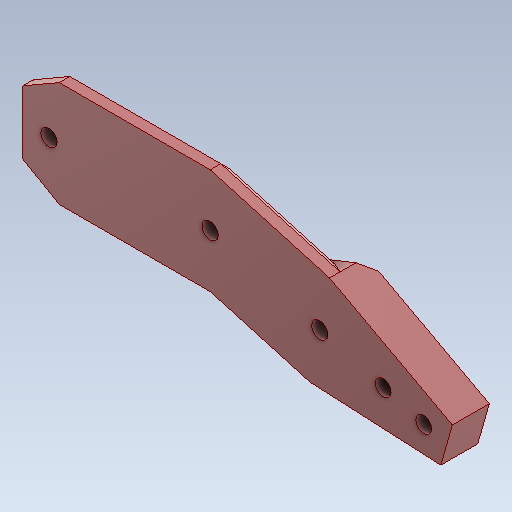
# Autodesk Inventor part: Fibula
Saved by Autodesk Inventor 2020 (Build 240168000, 168)
## iProperties
Created: 2020-09-15
Part Number: Fibula
Material: Generic
Document SubType Name: Modeling
Designer: Turing
Density: 1 g/cm^3
Appearance: Smooth - Burnt Red
Mass: 6.79509 g
Surface Area: 41.4305 cm^2
Volume: 6.79509 cm^3
Author: Turing
Autodesk Inventor part; units mm, degrees
ref_plane "YZ Plane" through (0, 0, 0) normal (1, 0, 0) x (0, 1, 0)
ref_plane "XZ Plane" through (0, 0, 0) normal (0, 1, 0) x (-1, 0, 0)
ref_plane "XY Plane" through (0, 0, 0) normal (0, 0, 1) x (1, 0, 0)
sketch "Sketch1" plane through (0, 0, 0) normal (0, 0, 1) x (1, 0, 0)
  circle A0 centre (0, 0) radius 1.55
  line L0 (0, 0) -> (30.548, 0)
  circle A1 centre (30.548, 0) radius 1.55
  line L1 (30.548, 0) -> (51.3166, -5.9278)
  circle A2 centre (51.3166, -5.9278) radius 1.55
  line L2 (0, 0) -> (-5, 0)
  line L3 (-5, 0) -> (-5, 6)
  line L4 (-5, 6) -> (1.9282, 10)
  line L5 (-5, 0) -> (-5, -6)
  line L6 (1.9282, 10) -> (30.548, 10)
  line L7 (-5, -6) -> (1.9282, -10)
  line L8 (1.9282, -10) -> (30.548, -10)
  line L9 (30.548, -10) -> (49.4624, -15.3986)
  line L10 (30.548, 10) -> (53.1707, 3.5429)
  line L11 (0, 0) -> (1.9282, 0)
  line L12 (51.3166, -5.9278) -> (75.3565, -12.7894)
  line L13 (75.3565, -12.7894) -> (76.4544, -8.943)
  line L14 (76.4544, -8.943) -> (53.1707, 3.5429)
  line L15 (75.3565, -12.7894) -> (74.2587, -16.6358)
  line L16 (49.4624, -15.3986) -> (74.2587, -16.6358)
  line L17 (51.3166, -5.9278) -> (75.3565, -12.7894)
  circle A3 centre (63.3366, -9.3586) radius 1.5
  line L18 (63.3366, -9.3586) -> (71.0293, -11.5543)
  circle A4 centre (71.0293, -11.5543) radius 1.5
  dimension "d0" = 3.1
  dimension "d1" = 30.548
  dimension "d2" = 3.1
  dimension "d3" = 164.07
  dimension "d4" = 3.1
  dimension "d5" = 21.598
  dimension "d6" = 5
  dimension "d7" = 6
  dimension "d8" = 6
  dimension "d9" = 120
  dimension "d10" = 8
  dimension "d11" = 120
  dimension "d12" = 8
  dimension "d13" = 28.6198
  dimension "d14" = 28.6198
  dimension "d15" = 19.6698
  dimension "d16" = 23.5262
  dimension "d23" = 1.9282
  dimension "d54" = 25
  dimension "d55" = 180
  dimension "d56" = 4
  dimension "d57" = 4
  dimension "d58" = 90
  dimension "d59" = 90
  dimension "d60" = 3
  dimension "d61" = 8
  dimension "d62" = 3
  constraints: 38 end point, 5 centre point, 4 coincident, 4 horizontal, 2 parallel, 2 point on line, 1 collinear, 1 midpoint, 1 perpendicular, 1 vertical
  measures "d0" diameter of A0
  measures "d1" distance of L0.start L0.end
  measures "d2" diameter of A1
  measures "d3" angle of L1 L0
  measures "d4" diameter of A2
  measures "d5" distance of L1.start L1.end
  measures "d6" distance of L0.start L2.end
  measures "d7" distance of L2.end L3.end
  measures "d8" distance of L2.end L5.end
  measures "d9" angle of L4 L3
  measures "d10" distance of L3.end L4.end
  measures "d11" angle of L7 L5
  measures "d12" distance of L5.end L7.end
  measures "d13" distance of L7.end L8.end
  measures "d14" distance of L4.end L6.end
  measures "d15" distance of L8.end L9.end
  measures "d16" distance of L6.end L10.end
  measures "d23" distance of L11.end point (0, 0)
  measures "d54" distance of L12.start L12.end
  measures "d55" angle of L12 L1
  measures "d56" distance of L12.end L13.end
  measures "d57" distance of L12.end L15.end
  measures "d58" angle of L12 L15
  measures "d59" angle of L13 L12
  measures "d60" diameter of A3
  measures "d61" distance of L18.start L18.end
  measures "d62" diameter of A4
extrude "Extrusion1" add sketch "Sketch1" along normal blind 4 contours L0 A1 L1 A2 L12 A3 A4 L15 L16 L9 L8 L7 L5 L2 A0 | A0 L2 L3 L4 L6 L10 L14 L13 L12 A4 A3 A2 L1 A1 L0
sketch "Sketch3" plane through (0, 0, 4) normal (0, 0, 1) x (1, 0, 0)
  line L0 (1.9282, -10) -> (30.548, -10) projected
  line L1 (30.548, -10) -> (49.4624, -15.3986) projected
  line L2 (49.4624, -15.3986) -> (74.2587, -16.6358) projected
  line L3 (74.2587, -16.6358) -> (76.4544, -8.943) projected
  line L4 (76.4544, -8.943) -> (53.1707, 3.5429) projected
  line L5 (53.1707, 3.5429) -> (30.548, 10) projected
  line L6 (30.548, 10) -> (1.9282, 10) projected
  line L7 (1.9282, 10) -> (-5, 6) projected
  line L8 (-5, 6) -> (-5, -6) projected
  line L9 (-5, -6) -> (1.9282, -10) projected
  circle A0 centre (71.0293, -11.5543) radius 1.5 projected
  circle A1 centre (63.3366, -9.3586) radius 1.5 projected
  circle A2 centre (51.3166, -5.9278) radius 1.55 projected
  circle A3 centre (30.548, 0) radius 1.55 projected
  circle A4 centre (0, 0) radius 1.55 projected
  line L10 (49.4624, -15.3986) -> (42.7525, -7.984)
  line L11 (42.7525, -7.984) -> (43.8857, -0.1703)
  line L12 (43.8857, -0.1703) -> (53.1707, 3.5429)
  dimension "d63" = 10
  dimension "d64" = 10
  dimension "d65" = 130
  dimension "d66" = 135
  constraints: 6 end point
  measures "d63" distance of L1.end L10.end
  measures "d64" distance of L11.end L4.end
  measures "d65" angle of L4 L12
  measures "d66" angle of L2 L10
extrude "Extrusion2" add sketch "Sketch3" against normal blind 7 contours L10 L11 L12 L4 L3 L2
sketch "Sketch4" plane through (0, 0, -3) normal (0, 0, -1) x (-1, 0, 0)
  line L0 (-53.1707, 3.5429) -> (-76.4544, -8.943) projected
  line L1 (-76.4544, -8.943) -> (-74.2587, -16.6358) projected
  line L2 (-74.2587, -16.6358) -> (-49.4624, -15.3986) projected
  line L3 (-49.4624, -15.3986) -> (-42.7525, -7.984) projected
  line L4 (-42.7525, -7.984) -> (-43.8857, -0.1703) projected
  line L5 (-43.8857, -0.1703) -> (-53.1707, 3.5429) projected
  circle A0 centre (-71.0293, -11.5543) radius 1.5 projected
  circle A1 centre (-51.3166, -5.9278) radius 1.55 projected
  circle A2 centre (-63.3366, -9.3586) radius 1.5 projected
  circle A3 centre (-71.0293, -11.5543) radius 2.8
  circle A4 centre (-63.3366, -9.3586) radius 2.8
  circle A5 centre (-51.3166, -5.9278) radius 2.8
  point P0 (0, 0)
  dimension "d69" = 5.6
  dimension "d70" = 5.6
  dimension "d71" = 5.6
  constraints: 3 centre point, 3 coincident
  measures "d69" diameter of A3
  measures "d70" diameter of A4
  measures "d71" diameter of A5
extrude "Extrusion3" cut sketch "Sketch4" against normal blind 2 contours A3 | A4 | A5
chamfer "Chamfer1" distance 2 angle 45 10 edges at (41.8594, 6.7715, 0) (16.2381, -10, 0) (40.0052, -12.6993, 0) (-1.5359, -8, 0) (-5, 0, 0) (-1.5359, 8, 0) (16.2381, 10, 0) (48.5282, 1.6863, -3) (43.3191, -4.0771, -3) (46.1075, -11.6913, -3)
equation "\"d8\" = d7"
equation "\"d11\" = d9"
equation "\"d12\" = d10"
equation "\"d13\" = d1 - d23"
equation "\"d14\" = d1 - d23"
equation "\"d15\" = d5 - d23"
equation "\"d16\" = d5 + d23"
equation "\"d57\" = d56"
equation "\"d58\" = d59"
equation "\"d70\" = d69"
equation "\"d71\" = d69"
body "Solid1"
